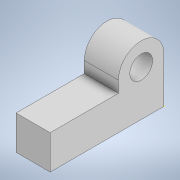
# Autodesk Inventor part: Suporte
Saved by Autodesk Inventor 2021 (Build 250183000, 183)
## iProperties
Created: 2022-02-01
Part Number: Suporte
Material: Genérico
Document SubType Name: Modeling
Designer: aluno
Density: 1 g/cm^3
Appearance: Padrão
Author: aluno
Autodesk Inventor part; units mm, degrees
ref_plane "YZ Plane" through (0, 0, 0) normal (1, 0, 0) x (0, 1, 0)
ref_plane "XZ Plane" through (0, 0, 0) normal (0, 1, 0) x (-1, 0, 0)
ref_plane "XY Plane" through (0, 0, 0) normal (0, 0, 1) x (1, 0, 0)
sketch "Esboço1" plane through (0, 0, 0) normal (1, 0, 0) x (0, 1, 0)
  line L0 (0, 0) -> (30, 0)
  line L1 (30, 0) -> (30, 100)
  line L2 (30, 100) -> (0, 100)
  line L3 (0, 100) -> (0, 0)
  dimension "d0" = 30
  dimension "d1" = 100
  constraints: 8 end point, 2 parallel, 1 horizontal, 1 perpendicular
  measures "d0" distance of L2.end L1.end
  measures "d1" distance of L1.end L0.end
extrude "Extrusão1" add sketch "Esboço1" against normal blind 30
sketch "Esboço2" plane through (0, 0, 0) normal (1, 0, 0) x (0, 0, -1)
  point P0 (0, 0)
sketch "Esboço3" plane through (0, 30, 100) normal (0, 1, 0) x (1, 0, 0)
  line L0 (-30, 0) -> (-30, 100) projected
  line L1 (0, 100) -> (0, 0) projected
  line L2 (-30, 100) -> (0, 100)
  line L3 (0, 100) -> (0, 60)
  line L4 (0, 60) -> (-30, 60)
  line L5 (-30, 60) -> (-30, 100)
  dimension "d4" = 40
  constraints: 8 end point, 2 parallel, 1 horizontal, 1 perpendicular, 1 point on line
  measures "d4" distance of L2.end L3.end
extrude "Extrusão2" add sketch "Esboço3" along normal blind 30
fillet "Arredondamento2" radius 20 2 edges at (-15, 60, 40) (-15, 60, 0)
sketch "Esboço6" plane through (0, 0, 0) normal (1, 0, 0) x (0, 0, -1)
  arc A0 (0, 40) -> (-40, 40) centre (-20, 40) ccw projected
  point P0 (0, 0)
  constraints: 1 coincident
hole "Furo3" at (0, 40, 20) direction (-1, 0, 0) diameter 20 end through all
